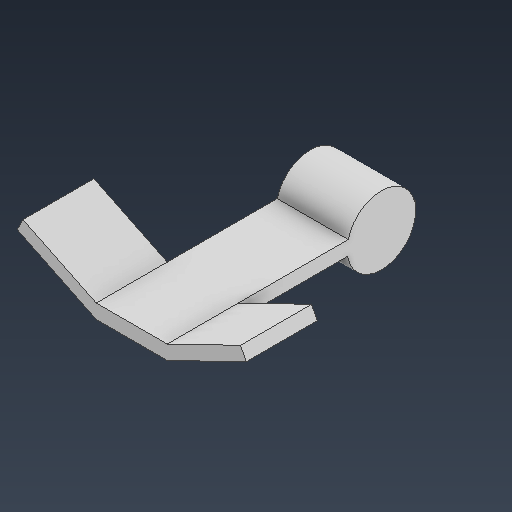
# Autodesk Inventor part: ПАЛЬЧИК
Saved by Autodesk Inventor 2026 (Build 300175000, 175)
## iProperties
Created: 2026-01-11
Part Number: ПАЛЬЧИК
Material: Типовые
Document SubType Name: Modeling
Designer: GameHD
Density: 1 g/cm^3
Appearance: По умолчанию
Author: GameHD
Autodesk Inventor part; units mm, degrees
ref_plane "YZ Plane" through (0, 0, 0) normal (1, 0, 0) x (0, 1, 0)
ref_plane "XZ Plane" through (0, 0, 0) normal (0, 1, 0) x (-1, 0, 0)
ref_plane "XY Plane" through (0, 0, 0) normal (0, 0, 1) x (1, 0, 0)
sketch "Эскиз1" plane through (0, 0, 0) normal (1, 0, 0) x (0, 1, 0)
  line L0 (0, 0) -> (4, 0)
  line L1 (4, 0) -> (4, -70)
  line L2 (4, -70) -> (0, -70)
  line L3 (0, -70) -> (0, 0)
  dimension "d0" = 4
  dimension "d1" = 70
  constraints: 8 end point, 2 parallel, 1 horizontal, 1 perpendicular
  measures "d0" distance of L1.end L2.end
  measures "d1" distance of L0.end L1.end
extrude "Выдавливание1" add sketch "Эскиз1" along normal blind 20
sketch "Эскиз2" plane through (0, 0, 0) normal (0, 0, 1) x (1, 0, 0)
  line L0 (0, 0) -> (0, 4) projected
  line L1 (0, 4) -> (-20.6542, 14.0196)
  line L2 (-20.6542, 14.0196) -> (-22.225, 10.7816)
  line L3 (-22.225, 10.7816) -> (0, 0)
  line L4 (0, 4) -> (20, 4) projected
  line L5 (0, 0) -> (20, 0) projected
  line L6 (10, 4) -> (10, 0)
  line L7 (20, 4) -> (40.6542, 14.0196)
  line L8 (40.6542, 14.0196) -> (42.225, 10.7816)
  line L9 (42.225, 10.7816) -> (20, 0)
  constraints: 14 end point, 2 midpoint, 2 symmetric about line, 1 parallel, 1 perpendicular
extrude "Выдавливание2" add sketch "Эскиз2" against normal blind 20 contours L3 L2 L1 L0 | L6 L4 L7 L8 L9 L5
sketch "Эскиз3" plane through (20, 0, 0) normal (1, 0, 0) x (0, 0, -1)
  circle A0 centre (60.325, 1.5875) radius 9.6564
  point P0 (0, 0)
  constraints: 1 centre point
extrude "Выдавливание3" add sketch "Эскиз3" against normal blind 20
